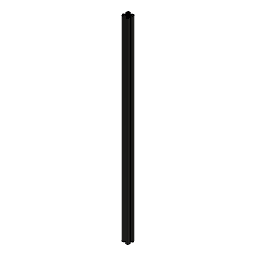
2020+v4 (Autodesk Fusion 360 design; units mm, degrees)
Autodesk Fusion 360 part; units mm, degrees
sketch "Sketch2" plane through (0, 0, 0) normal (0, 0, 1) x (1, 0, 0) in component "Component"
  circle A0 centre (0, 0) radius 2.15
  line L0 (-3.4043, 4.4638) -> (-5.5732, 6.8378)
  line L1 (-4.9826, 8.1774) -> (-3, 8.1774)
  line L2 (-2.5, 8.6774) -> (-2.5, 9.5)
  line L3 (-3, 10) -> (-8, 10)
  line L4 (-10, 8) -> (-10, 3)
  line L5 (-9.5, 2.5) -> (-8.7, 2.5)
  line L6 (-8.2, 3) -> (-8.2, 4.9826)
  line L7 (-6.8094, 5.5222) -> (-4.3043, 2.7802)
  arc A1 (-8, 10) -> (-10, 8) centre (-8, 8) ccw
  arc A2 (-2.5, 9.5) -> (-3, 10) centre (-3, 9.5) ccw
  arc A3 (-10, 3) -> (-9.5, 2.5) centre (-9.5, 3) ccw
  arc A4 (-8.7, 2.5) -> (-8.2, 3) centre (-8.7, 3) ccw
  arc A5 (-6.8094, 5.5222) -> (-8.2, 4.9826) centre (-7.4, 4.9826) ccw
  arc A6 (-4.9826, 8.1774) -> (-5.5732, 6.8378) centre (-4.9826, 7.3774) ccw
  arc A7 (-3, 8.1774) -> (-2.5, 8.6774) centre (-3, 8.6774) ccw
  line L8 (-1.5586, 3.65) -> (0.9669, 3.65)
  arc A8 (-3.4043, 4.4638) -> (-1.5586, 3.65) centre (-1.5586, 6.15) ccw
  arc A9 (-4.8251, -3.6514) -> (-3.65, -1.4406) centre (-6.0873, -1.5628) ccw
  arc A10 (-8.2009, -3.0209) -> (-8.7005, -2.5) centre (-8.7005, -3) ccw
  arc A11 (-3, -10) -> (-2.5, -9.5) centre (-3, -9.5) ccw
  arc A12 (-9.5, -2.5) -> (-10, -3) centre (-9.5, -3) ccw
  line L9 (-2.5, -9.5) -> (-2.5, -8.7)
  line L10 (-10, -3) -> (-10, -8)
  line L11 (-8.7005, -2.5) -> (-9.5, -2.5)
  arc A13 (-2.5, -8.7) -> (-3, -8.2) centre (-3, -8.7) ccw
  line L12 (-4.8251, -3.6514) -> (-7.1291, -5.7563)
  line L13 (-3.65, -1.4406) -> (-3.65, 1.094)
  line L14 (-3, -8.2) -> (-4.9826, -8.2)
  arc A14 (-8.2005, -5.0035) -> (-7.1291, -5.7563) centre (-7.4005, -5.0037) ccw
  arc A15 (-5.5222, -6.8094) -> (-4.9826, -8.2) centre (-4.9826, -7.4) ccw
  line L15 (-8, -10) -> (-3, -10)
  line L16 (-8.2005, -5.0035) -> (-8.2009, -3.0209)
  line L17 (-5.5222, -6.8094) -> (-2.7802, -4.3043)
  arc A16 (3.2759, -4.3232) -> (1.4298, -3.65) centre (1.5824, -6.0993) ccw
  arc A17 (3.0209, -8.2009) -> (2.5, -8.7005) centre (3, -8.7005) ccw
  arc A18 (10, -3) -> (9.5, -2.5) centre (9.5, -3) ccw
  arc A19 (2.5, -9.5) -> (3, -10) centre (3, -9.5) ccw
  line L18 (9.5, -2.5) -> (8.7, -2.5)
  line L19 (3, -10) -> (8, -10)
  line L20 (2.5, -8.7005) -> (2.5, -9.5)
  arc A20 (8.7, -2.5) -> (8.2, -3) centre (8.7, -3) ccw
  arc A21 (8, -10) -> (10, -8) centre (8, -8) ccw
  line L21 (3.2759, -4.3232) -> (5.5943, -6.8609)
  line L22 (1.4298, -3.65) -> (-1.094, -3.65)
  line L23 (8.2, -3) -> (8.2, -4.9826)
  arc A22 (5.0035, -8.2005) -> (5.5943, -6.8609) centre (5.0037, -7.4005) ccw
  arc A23 (6.8094, -5.5222) -> (8.2, -4.9826) centre (7.4, -4.9826) ccw
  line L24 (10, -8) -> (10, -3)
  line L25 (5.0035, -8.2005) -> (3.0209, -8.2009)
  line L26 (6.8094, -5.5222) -> (4.3043, -2.7802)
  arc A24 (4.3232, 3.2759) -> (3.65, 1.4298) centre (6.0993, 1.5824) ccw
  arc A25 (8.2009, 3.0209) -> (8.7005, 2.5) centre (8.7005, 3) ccw
  arc A26 (3, 10) -> (2.5, 9.5) centre (3, 9.5) ccw
  arc A27 (9.5, 2.5) -> (10, 3) centre (9.5, 3) ccw
  line L27 (2.5, 9.5) -> (2.5, 8.7)
  line L28 (10, 3) -> (10, 8)
  line L29 (8.7005, 2.5) -> (9.5, 2.5)
  arc A28 (2.5, 8.7) -> (3, 8.2) centre (3, 8.7) ccw
  arc A29 (10, 8) -> (8, 10) centre (8, 8) ccw
  line L30 (4.3232, 3.2759) -> (6.8609, 5.5943)
  line L31 (3.65, 1.4298) -> (3.65, -1.094)
  line L32 (3, 8.2) -> (4.9826, 8.2)
  arc A30 (8.2005, 5.0035) -> (6.8609, 5.5943) centre (7.4005, 5.0037) ccw
  arc A31 (5.4644, 6.8727) -> (4.9826, 8.2) centre (4.9591, 7.4404) ccw
  line L33 (8, 10) -> (3, 10)
  line L34 (8.2005, 5.0035) -> (8.2009, 3.0209)
  line L35 (5.4644, 6.8727) -> (2.6531, 4.3043)
  arc A32 (0.9669, 3.65) -> (2.6531, 4.3043) centre (0.9669, 6.15) ccw
  arc A33 (3.65, -1.094) -> (4.3043, -2.7802) centre (6.15, -1.094) ccw
  arc A34 (-1.094, -3.65) -> (-2.7802, -4.3043) centre (-1.094, -6.15) ccw
  arc A35 (-3.65, 1.094) -> (-4.3043, 2.7802) centre (-6.15, 1.094) ccw
  arc A36 (-10, -8) -> (-8, -10) centre (-8, -8) ccw
  point P0 (-10, 10)
  point P1 (-10, 2.5)
  point P2 (-10, -7.3311)
  point P3 (-8, -10)
  point P4 (-10, -10)
  point P5 (-2.5, -10)
  point P6 (10, -10)
  point P7 (10, -2.5)
  point P8 (10, 10)
  point P9 (2.5, 10)
  dimension "d17" = 4.3
  dimension "d18" = 2
  dimension "d22" = 0.5
  dimension "d23" = 0.5
  dimension "d24" = 0.5
  dimension "d25" = 1.8
  dimension "d26" = 0.8
  dimension "d27" = 0.8
  dimension "d28" = 0.5
  dimension "d39" = 1.8
  dimension "d40" = 2.5
  dimension "d43" = 2.5
  dimension "d44" = 2.5
  dimension "d45" = 2.5
  dimension "d46" = 2.5
  dimension "d47" = 5
  dimension "d48" = 6.35
  dimension "d49" = 20
  dimension "d50" = 20
  dimension "d51" = 6.35
  dimension "d52" = 6.35
  dimension "d53" = 6.35
  dimension "d54" = 2
  constraint coincident A0.centre origin
  constraint horizontal L1
  constraint perpendicular L1 L2
  constraint perpendicular L2 L3
  constraint perpendicular L1 L4
  constraint perpendicular L2 L5
  constraint perpendicular L5 L6
  constraint coincident P0 L4
  constraint coincident P0 L3
  constraint tangent L4 A1
  constraint tangent L3 A1
  constraint tangent L3 A2
  constraint tangent L2 A2
  constraint coincident P1 L4
  constraint coincident P1 L5
  constraint tangent L4 A3
  constraint tangent L5 A3
  constraint tangent L5 A4
  constraint tangent L6 A4
  constraint tangent L7 A5
  constraint tangent L6 A5
  constraint tangent L0 A6
  constraint tangent L1 A6
  constraint tangent L1 A7
  constraint tangent L2 A7
  constraint parallel L0 L7
  constraint horizontal L8
  constraint tangent L0 A8
  constraint tangent L8 A8
  constraint tangent L8 A32
  constraint tangent L35 A32
  constraint tangent L31 A33
  constraint tangent L26 A33
  constraint tangent L22 A34
  constraint tangent L17 A34
  constraint tangent L13 A35
  constraint tangent L7 A35
  constraint vertical L31
  constraint horizontal L22
  constraint horizontal L15
  constraint collinear L15 L19
  constraint collinear L4 L10
  constraint collinear L24 L28
  constraint coincident P2 L10
  constraint coincident P3 L15
  constraint tangent L10 A36
  constraint tangent L15 A36
  constraint collinear L3 L33
  constraint vertical L13
  constraint parallel L12 L17
  constraint parallel L21 L26
  constraint parallel L30 L35
  constraint equal L1 L6
  constraint equal L1 L32
  constraint equal L32 L34
  constraint equal L23 L34
  constraint equal L23 L25
  constraint equal L14 L16
  measures "d17" diameter of A0
  measures "d18" radius of A1
  measures "d22" radius of A2
  measures "d23" radius of A3
  measures "d24" radius of A4
  measures "d25" distance of L4.end L6.start
  measures "d26" radius of A5
  measures "d27" radius of A6
  measures "d28" radius of A7
  measures "d39" distance of L0 L7
  measures "d40" radius of A8
  measures "d43" radius of A32
  measures "d44" radius of A33
  measures "d45" radius of A34
  measures "d46" radius of A35
  measures "d47" distance of A11.end A19.start
  measures "d48" vertical distance of P3 L22.end
  measures "d49" distance of L19.end A29.end
  measures "d50" distance of L4.start L28.end
  measures "d51" vertical distance of A29.end L8.end
  measures "d52" distance of A21.end L31
  measures "d53" horizontal distance of A9.end P2
  measures "d54" radius of A36
extrude "Extrude1" add sketch "Sketch2" along normal blind 600 in component "Component"
component "Component" placed x (1, 0, 0) y (0, 1, 0) z (0, 0, 1) at (0, 0, 0)
